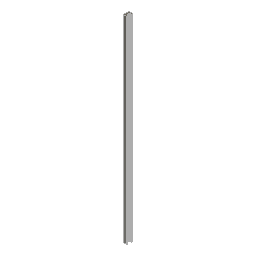
Боковое крепление хотвилс карточки (Autodesk Fusion 360 design; units mm, degrees)
Autodesk Fusion 360 part; units mm, degrees
sketch "Sketch1" plane through (0, 0, 0) normal (0, 0, 1) x (1, 0, 0)
  line L0 (0, -1.5) -> (0, 1.5)
  line L1 (0, 1.5) -> (2, 1.5)
  line L2 (2, 1.5) -> (2, 3)
  line L3 (2, 3) -> (-2, 3)
  line L4 (-2, 3) -> (-2, -3)
  line L5 (0, -1.5) -> (2, -1.5)
  line L6 (2, -3) -> (-2, -3)
  line L7 (2, -1.5) -> (2, -3)
  constraint vertical L0
  constraint perpendicular L0 L1
  constraint perpendicular L1 L2
  constraint perpendicular L2 L3
  constraint perpendicular L3 L4
extrude "Extrude1" add sketch "Sketch1" along normal blind 220
fillet "Fillet1" radius 0.5 8 edges at (2, -3, 110) (-2, -3, 110) (2, -1.5, 110) (0, -1.5, 110) (0, 1.5, 110) (2, 1.5, 110) (2, 3, 110) (-2, 3, 110)
